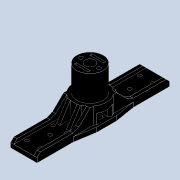
# Autodesk Inventor part: Axis 4 Male Bearing Connector Bracket
Saved by Autodesk Inventor 2022 (Build 260153000, 153)
## iProperties
Created: 2021-12-24
Part Number: Axis 4 Male Bearing Connector Bracket
Material: Generic
Document SubType Name: Modeling
Designer: Coy
Density: 1 g/cm^3
Appearance: Anodized - Black
Author: Coy
Autodesk Inventor part; units mm, degrees
ref_plane "YZ Plane" through (0, 0, 0) normal (1, 0, 0) x (0, 1, 0)
ref_plane "XZ Plane" through (0, 0, 0) normal (0, 1, 0) x (-1, 0, 0)
sketch "Sketch1" plane through (0, 0, 0) normal (0, 1, 0) x (-1, 0, 0)
  line L0 (0, 0) -> (40, 0)
  line L1 (40, 0) -> (40, 200)
  line L2 (40, 200) -> (0, 200)
  line L3 (0, 200) -> (0, 0)
  dimension "d0" = 200
  dimension "d1" = 40
  constraints: 8 end point, 2 parallel, 1 horizontal, 1 perpendicular
  measures "d0" distance of L0.end L1.end
  measures "d1" distance of L0.start L0.end
extrude "Extrusion1" add sketch "Sketch1" along normal blind 7
sketch "Sketch2" plane through (0, 0, 0) normal (0, -1, 0) x (1, 0, 0)
  line L0 (0, 200) -> (0, 0) construction
  line L1 (0, 100) -> (-40, 100) construction
  line L2 (-40, 0) -> (-40, 200) construction
  circle A0 centre (-20, 100) radius 20 construction
  line L3 (-40, 200) -> (0, 200) construction
  line L4 (-20, 200) -> (-20, 0) construction
  line L5 (0, 0) -> (-40, 0) construction
  line L6 (-9.65, 200) -> (-9.65, 0)
  line L7 (-30.35, 200) -> (-30.35, 0)
  line L8 (-9.65, 90) -> (-30.35, 90)
  line L9 (-30.35, 90) -> (-30.35, 23) construction
  line L10 (-30.35, 23) -> (-9.65, 23)
  line L11 (-9.65, 23) -> (-9.65, 90) construction
  line L12 (-9.65, 110) -> (-30.35, 110)
  line L13 (-30.35, 110) -> (-30.35, 177) construction
  line L14 (-30.35, 177) -> (-9.65, 177)
  line L15 (-9.65, 177) -> (-9.65, 110) construction
  line L16 (-9.65, 113.2) -> (-30.35, 113.2) construction
  line L17 (-9.65, 86.8) -> (-30.35, 86.8) construction
  point P0 (-9.65, 177)
  dimension "d19" = 1.25
  dimension "d4" = 40
  dimension "d5" = 10.35
  dimension "d6" = 10.35
  dimension "d7" = 67
  dimension "d8" = 67
  dimension "d9" = 3.2
  dimension "d10" = 3.2
  dimension "d11" = 20
  dimension "d12" = 10
  constraints: 28 end point, 8 point on line, 6 parallel, 5 midpoint, 4 perpendicular, 2 horizontal, 1 centre point
  measures "d4" diameter of A0
  measures "d5" distance between parallel lines of L4 L6
  measures "d6" distance between parallel lines of L4 L7
  measures "d7" distance of L9.end L8.end
  measures "d8" distance between parallel lines of L14 L12
  measures "d9" distance between parallel lines of L12 L16
  measures "d10" distance between parallel lines of L8 L17
  measures "d11" distance between parallel lines of L8 L12
  measures "d12" distance from line of A0.centre L12
extrude "Extrusion2" cut sketch "Sketch2" against normal blind 3.2 contours L6 L12 L7 L14 | L6 L10 L7 L8
sketch "Sketch3" plane through (0, 3.2, 0) normal (0, -1, 0) x (1, 0, 0)
  line L0 (-9.65, 177) -> (-9.65, 110) projected
  line L1 (-30.35, 110) -> (-30.35, 177) projected
  line L2 (-9.65, 110) -> (-30.35, 110)
  line L3 (-30.35, 110) -> (-30.35, 113.3)
  line L4 (-30.35, 113.3) -> (-9.65, 113.3)
  line L5 (-9.65, 113.3) -> (-9.65, 110)
  line L6 (-30.35, 90) -> (-9.65, 90) projected
  line L7 (-30.35, 23) -> (-30.35, 90) projected
  line L8 (-9.65, 90) -> (-30.35, 90)
  line L9 (-30.35, 90) -> (-30.35, 86.7)
  line L10 (-30.35, 86.7) -> (-9.65, 86.7)
  line L11 (-9.65, 86.7) -> (-9.65, 90)
  line L12 (-30.35, 177) -> (-9.65, 177) construction
  line L13 (-20, 177) -> (-20, 110) construction
  line L14 (-20, 90) -> (-20, 23) construction
  line L15 (-9.65, 23) -> (-30.35, 23) construction
  circle A0 centre (-20, 160) radius 2.65
  circle A1 centre (-20, 131) radius 2.65
  circle A2 centre (-20, 69) radius 2.65
  circle A3 centre (-20, 40) radius 2.65
  point P0 (0, 0)
  dimension "d15" = 3.3
  dimension "d16" = 3.3
  dimension "d20" = 5.3
  dimension "d21" = 5.3
  dimension "d22" = 5.3
  dimension "d23" = 5.3
  dimension "d24" = 29
  dimension "d25" = 29
  dimension "d26" = 21
  dimension "d27" = 21
  constraints: 20 end point, 6 point on line, 4 centre point, 4 midpoint, 4 parallel, 2 horizontal, 2 perpendicular
  measures "d15" distance of L2.end L3.end
  measures "d16" distance of L9.end L8.end
  measures "d20" diameter of A0
  measures "d21" diameter of A1
  measures "d22" diameter of A2
  measures "d23" diameter of A3
  measures "d24" distance of A1.centre A0.centre
  measures "d25" distance of A3.centre A2.centre
  measures "d26" distance from line of L2 A1.centre
  measures "d27" distance from line of L6 A2.centre
extrude "Extrusion3" cut sketch "Sketch3" against normal up to next
fillet "Fillet1" radius 1.25 2 edges at (-20, 3.2, 113.3) (-20, 3.2, 86.7)
sketch "Sketch4" plane through (0, 7, 0) normal (0, 1, 0) x (1, 0, 0)
  line L0 (-40, -200) -> (0, -200) construction
  line L1 (-30, -200) -> (-30, 0) construction
  line L2 (-40, 0) -> (-40, -200) construction
  circle A0 centre (-30, -185) radius 2.65
  circle A1 centre (-30, -145.5) radius 2.65
  circle A2 centre (-30, -54.5) radius 2.65
  circle A3 centre (-30, -15) radius 2.65
  line L3 (0, 0) -> (-40, 0) projected
  circle A4 centre (-20, -131) radius 2.65 projected
  circle A5 centre (-20, -69) radius 2.65 projected
  line L4 (-20, -200) -> (-20, 0) construction
  line L5 (0, 0) -> (-40, 0) construction
  line L6 (-10, -200) -> (-10, 0) construction
  line L7 (0, 0) -> (0, -200) construction
  circle A6 centre (-10, -185) radius 2.65
  circle A7 centre (-10, -145.5) radius 2.65
  circle A8 centre (-10, -54.5) radius 2.65
  circle A9 centre (-10, -15) radius 2.65
  dimension "d28" = 10
  dimension "d29" = 5.3
  dimension "d30" = 5.3
  dimension "d31" = 5.3
  dimension "d32" = 5.3
  dimension "d33" = 15
  dimension "d34" = 15
  dimension "d35" = 14.5
  dimension "d36" = 14.5
  constraints: 9 point on line, 8 centre point, 8 end point, 6 symmetric about line, 2 midpoint, 1 vertical, 4 other
  measures "d28" distance between parallel lines of L2 L1
  measures "d29" diameter of A0
  measures "d30" diameter of A1
  measures "d31" diameter of A2
  measures "d32" diameter of A3
  measures "d33" distance from line of L0 A0.centre
  measures "d34" distance from line of L3 A3.centre
  measures "d35" vertical distance of A4.centre A1.centre
  measures "d36" vertical distance of A5.centre A2.centre
extrude "Extrusion4" cut sketch "Sketch4" against normal up to next contours A0 | A1 | A2 | A3 | A6 | A7 | A8 | A9
sketch "Sketch5" plane through (0, 7, 0) normal (0, 1, 0) x (1, 0, 0)
  circle A0 centre (-30, -145.5) radius 2.65 projected
  circle A1 centre (-30, -15) radius 2.65 projected
  circle A2 centre (-10, -54.5) radius 2.65 projected
  circle A3 centre (-10, -185) radius 2.65 projected
  circle A4 centre (-10, -145.5) radius 2.65 projected
  circle A5 centre (-10, -15) radius 2.65 projected
  circle A6 centre (-30, -54.5) radius 2.65 projected
  circle A7 centre (-30, -185) radius 2.65 projected
  circle A8 centre (-20, -69) radius 2.65 projected
  line L0 (-30.35, -90) -> (-30.35, -86.7) projected
  line L1 (-30.35, -86.7) -> (-9.65, -86.7) projected
  line L2 (-9.65, -86.7) -> (-9.65, -90) projected
  line L3 (-9.65, -90) -> (-30.35, -90) projected
  circle A9 centre (-20, -131) radius 2.65 projected
  circle A10 centre (-20, -40) radius 2.65 projected
  line L4 (-9.65, -113.3) -> (-30.35, -113.3) projected
  line L5 (-30.35, -113.3) -> (-30.35, -110) projected
  line L6 (-30.35, -110) -> (-9.65, -110) projected
  line L7 (-9.65, -110) -> (-9.65, -113.3) projected
  circle A11 centre (-20, -160) radius 2.65 projected
  line L8 (-40, 0) -> (-40, -200) projected
  line L9 (-40, -200) -> (0, -200) projected
  line L10 (0, -200) -> (0, 0) projected
  line L11 (0, 0) -> (-40, 0) projected
  line L12 (-40, -200) -> (0, -200) construction
  line L13 (-20, -200) -> (-20, 0) construction
  line L14 (0, 0) -> (-40, 0) construction
  circle A12 centre (-20, -100) radius 20
  line L15 (-40, 0) -> (-40, -200) projected
  circle A13 centre (-20, -100) radius 7.5
  dimension "d39" = 15
  constraints: 3 midpoint, 2 centre point, 2 end point, 1 coincident, 1 tangent
  measures "d39" diameter of A13
extrude "Extrusion5" add sketch "Sketch5" along normal blind 64 contours A12
sketch "Sketch6" plane through (0, 7, 0) normal (0, 1, 0) x (1, 0, 0)
  circle A0 centre (-20, -69) radius 2.65 construction
  circle A1 centre (-20, -69) radius 5 construction
  circle A2 centre (-20, -100) radius 20 projected
  circle A3 centre (-20, -100) radius 25
  point P0 (0, 0)
  dimension "d42" = 10
  dimension "d43" = 50
  constraints: 2 centre point, 2 coincident
  measures "d42" diameter of A1
  measures "d43" diameter of A3
extrude "Extrusion6" add sketch "Sketch6" along normal blind 25
sketch "Sketch7" plane through (-20, 71, 100) normal (0, 1, 0) x (1, 0, 0)
  line L0 (-20, 15) -> (-20, -15) construction
  line L1 (-20, 0) -> (20, 0) construction
  circle A0 centre (0, 0) radius 20 construction
  circle A1 centre (-13.75, 0) radius 2.75
  circle A2 centre (13.75, 0) radius 2.75
  circle A3 centre (-13.75, 0) radius 5 construction
  circle A4 centre (13.75, 0) radius 5 construction
  point P0 (20, 100)
  dimension "d46" = 5.5
  dimension "d47" = 5.5
  dimension "d48" = 6.25
  dimension "d49" = 10
  dimension "d50" = 10
  dimension "d51" = 6.25
  constraints: 4 centre point, 2 coincident, 2 end point, 2 point on line, 1 horizontal, 1 midpoint, 1 point on circle
  measures "d46" diameter of A1
  measures "d47" diameter of A2
  measures "d48" distance of L1.start A1.centre
  measures "d49" diameter of A3
  measures "d50" diameter of A4
  measures "d51" distance of L1.end A2.centre
extrude "Extrusion7" cut sketch "Sketch7" against normal up to next
sketch "Sketch8" plane through (0, 0, 0) normal (0, -1, 0) x (1, 0, 0)
  circle A0 centre (-6.25, 100) radius 2.75 projected
  circle A1 centre (-33.75, 100) radius 2.75 projected
  line L0 (-2.25, 97.6906) -> (-6.25, 95.3812)
  line L1 (-6.25, 95.3812) -> (-10.25, 97.6906)
  line L2 (-10.25, 97.6906) -> (-10.25, 102.3094)
  line L3 (-10.25, 102.3094) -> (-6.25, 104.6188)
  line L4 (-6.25, 104.6188) -> (-2.25, 102.3094)
  line L5 (-2.25, 102.3094) -> (-2.25, 97.6906)
  line L6 (-29.75, 97.6906) -> (-33.75, 95.3812)
  line L7 (-33.75, 95.3812) -> (-37.75, 97.6906)
  line L8 (-37.75, 97.6906) -> (-37.75, 102.3094)
  line L9 (-37.75, 102.3094) -> (-33.75, 104.6188)
  line L10 (-33.75, 104.6188) -> (-29.75, 102.3094)
  line L11 (-29.75, 102.3094) -> (-29.75, 97.6906)
  point P0 (0, 0)
  dimension "d54" = 8
  dimension "d55" = 8
  constraints: 24 end point, 2 coincident, 26 other
  measures "d54" distance between parallel lines of L2 L5
  measures "d55" distance between parallel lines of L8 L11
extrude "Extrusion8" cut sketch "Sketch8" against normal blind 51
sketch "Sketch9" plane through (0, 0, 0) normal (0, -1, 0) x (1, 0, 0)
  line L0 (-37.75, 102.3094) -> (-33.75, 104.6188) projected
  line L1 (-33.75, 104.6188) -> (-29.75, 102.3094) projected
  line L2 (-29.75, 102.3094) -> (-29.75, 97.6906) projected
  line L3 (-29.75, 97.6906) -> (-33.75, 95.3812) projected
  line L4 (-33.75, 95.3812) -> (-37.75, 97.6906) projected
  line L5 (-37.75, 97.6906) -> (-37.75, 102.3094) projected
  line L6 (-10.25, 102.3094) -> (-6.25, 104.6188) projected
  line L7 (-6.25, 104.6188) -> (-2.25, 102.3094) projected
  line L8 (-2.25, 102.3094) -> (-2.25, 97.6906) projected
  line L9 (-2.25, 97.6906) -> (-6.25, 95.3812) projected
  line L10 (-6.25, 95.3812) -> (-10.25, 97.6906) projected
  line L11 (-10.25, 97.6906) -> (-10.25, 102.3094) projected
  line L12 (-40, 0) -> (-40, 200) projected
  line L13 (0, 0) -> (-40, 0) projected
  line L14 (0, 200) -> (0, 0) projected
  line L15 (-40, 200) -> (0, 200) projected
  arc A0 (-9.65, 51.8732) -> (-9.65, 57.1268) centre (-10, 54.5) ccw projected
  line L16 (-9.65, 51.8732) -> (-9.65, 23) projected
  line L17 (-9.65, 23) -> (-30.35, 23) projected
  line L18 (-30.35, 23) -> (-30.35, 51.8732) projected
  arc A1 (-30.35, 57.1268) -> (-30.35, 51.8732) centre (-30, 54.5) ccw projected
  line L19 (-30.35, 57.1268) -> (-30.35, 90) projected
  line L20 (-30.35, 90) -> (-9.65, 90) projected
  line L21 (-9.65, 90) -> (-9.65, 57.1268) projected
  circle A2 centre (-30, 185) radius 2.65 projected
  circle A3 centre (-10, 15) radius 2.65 projected
  circle A4 centre (-10, 185) radius 2.65 projected
  circle A5 centre (-30, 15) radius 2.65 projected
  arc A6 (-30.35, 148.1268) -> (-30.35, 142.8732) centre (-30, 145.5) ccw projected
  line L22 (-30.35, 148.1268) -> (-30.35, 177) projected
  line L23 (-30.35, 177) -> (-9.65, 177) projected
  line L24 (-9.65, 177) -> (-9.65, 148.1268) projected
  arc A7 (-9.65, 142.8732) -> (-9.65, 148.1268) centre (-10, 145.5) ccw projected
  line L25 (-9.65, 142.8732) -> (-9.65, 110) projected
  line L26 (-9.65, 110) -> (-30.35, 110) projected
  line L27 (-30.35, 110) -> (-30.35, 142.8732) projected
  line L28 (0, 115) -> (0, 85) projected
  arc A8 (0, 85) -> (0, 115) centre (-20, 100) ccw projected
  line L29 (-40, 85) -> (-40, 115) projected
  arc A9 (-40, 115) -> (-40, 85) centre (-20, 100) ccw projected
  line L30 (5, 115) -> (-45, 115)
  line L31 (-45, 115) -> (-45, 85)
  line L32 (-45, 85) -> (5, 85)
  line L33 (5, 85) -> (5, 115)
  line L34 (5, 115) -> (0, 145.5)
  line L35 (0, 200) -> (0, 0) projected
  line L36 (-45, 115) -> (-40, 145.5)
  line L37 (-40, 0) -> (-40, 200) projected
  line L38 (-45, 85) -> (-40, 54.5)
  line L39 (5, 85) -> (0, 54.5)
  constraints: 16 end point, 4 parallel, 4 point on line, 1 horizontal, 1 perpendicular
extrude "Extrusion9" add sketch "Sketch9" against normal up to surface (7 mm away) contours L38 L32 L12 | A9 L12 | L32 L31 A9 | L14 L32 L39 | L30 L36 L12 | A9 L31 L30 | L14 A8 | A8 L33 L32 | L30 L33 A8 | L14 L34 L30
sketch "Sketch10" plane through (0, 7, 0) normal (0, 1, 0) x (1, 0, 0)
  arc A0 (-45, -100) -> (5, -100) centre (-20, -100) ccw projected
  line L0 (-45, -115) -> (-45, -100) projected
  line L1 (-40, -145.5) -> (-45, -115) projected
  line L2 (-40, -145.5) -> (-40, -200) projected
  line L3 (-40, -200) -> (0, -200) projected
  line L4 (0, -200) -> (0, -145.5) projected
  line L5 (5, -115) -> (0, -145.5) projected
  line L6 (5, -100) -> (5, -115) projected
  circle A1 centre (-20, -160) radius 2.65 projected
  circle A2 centre (-20, -131) radius 2.65 projected
  circle A3 centre (-30, -185) radius 2.65 projected
  circle A4 centre (-10, -145.5) radius 2.65 projected
  circle A5 centre (-10, -185) radius 2.65 projected
  circle A6 centre (-30, -145.5) radius 2.65 projected
  circle A7 centre (-20, -40) radius 2.65 projected
  circle A8 centre (-20, -69) radius 2.65 projected
  circle A9 centre (-30, -54.5) radius 2.65 projected
  circle A10 centre (-10, -15) radius 2.65 projected
  circle A11 centre (-10, -54.5) radius 2.65 projected
  circle A12 centre (-30, -15) radius 2.65 projected
  arc A13 (5, -100) -> (-45, -100) centre (-20, -100) ccw projected
  line L7 (5, -85) -> (5, -100) projected
  line L8 (0, -54.5) -> (5, -85) projected
  line L9 (0, -54.5) -> (0, 0) projected
  line L10 (0, 0) -> (-40, 0) projected
  line L11 (-40, 0) -> (-40, -54.5) projected
  line L12 (-45, -85) -> (-40, -54.5) projected
  line L13 (-45, -100) -> (-45, -85) projected
  line L14 (-65.195, -100) -> (40.5448, -100) construction
  circle A14 centre (-10, -145.5) radius 5 construction
  line L15 (5, -115) -> (0, -145.5) projected
  line L16 (0, -145.5) -> (-5, -145.5)
  line L17 (-5, -145.5) -> (-5, -120)
  arc A15 (-45, -100) -> (5, -100) centre (-20, -100) ccw projected
  line L18 (0, -200) -> (0, -145.5) projected
  line L19 (0, -145.5) -> (0, -115)
  line L20 (-40, -200) -> (0, -200) construction
  line L21 (-20, -200) -> (-20, 0) construction
  line L22 (0, 0) -> (-40, 0) construction
  circle A16 centre (-20, -131) radius 2.65 construction
  circle A17 centre (-20, -131) radius 5 construction
  line L23 (-15, -124.4949) -> (-15, -140.5)
  line L24 (-15, -140.5) -> (-10, -140.5)
  line L25 (-10, -140.5) -> (-10, -122.9129)
  line L26 (-40, -145.5) -> (-35, -145.5)
  line L27 (-35, -145.5) -> (-35, -120)
  line L28 (-40, -145.5) -> (-40, -115)
  line L29 (-25, -124.4949) -> (-25, -140.5)
  line L30 (-25, -140.5) -> (-30, -140.5)
  line L31 (-30, -140.5) -> (-30, -122.9129)
  line L32 (0, -54.5) -> (-5, -54.5)
  line L33 (-5, -54.5) -> (-5, -80)
  line L34 (0, -54.5) -> (0, -85)
  line L35 (-15, -75.5051) -> (-15, -59.5)
  line L36 (-15, -59.5) -> (-10, -59.5)
  line L37 (-10, -59.5) -> (-10, -77.0871)
  line L38 (-25, -75.5051) -> (-25, -59.5)
  line L39 (-25, -59.5) -> (-30, -59.5)
  line L40 (-30, -59.5) -> (-30, -77.0871)
  line L41 (-35, -54.5) -> (-35, -80)
  line L42 (-40, -54.5) -> (-35, -54.5)
  line L43 (-40, -54.5) -> (-40, -85)
  dimension "d60" = 10
  dimension "d61" = 5
  dimension "d62" = 10
  dimension "d63" = 5
  constraints: 52 end point, 21 symmetric about line, 6 point on circle, 2 centre point, 2 coincident, 2 midpoint, 2 perpendicular, 1 collinear, 1 vertical
  measures "d60" diameter of A14
  measures "d61" distance of L4.end L16.end
  measures "d62" diameter of A17
  measures "d63" distance of L23.end L24.end
extrude "Extrusion10" add sketch "Sketch10" along normal blind 25 contours A0 L27 L26 L28 | L43 L42 L41 A13 | A0 L29 L30 L31 | L40 L39 L38 A13 | A0 L25 L24 L23 | L16 L17 A0 L19 | L35 L36 L37 A13 | L34 A13 L33 L32
chamfer "Chamfer1" distance 25.5 distance2 25 1 edges at (-2.5, 32, 145.5) measured on face at (-38.3333, 32, 126.8333)
chamfer "Chamfer2" distance 25.5 distance2 25 1 edges at (-37.5, 32, 145.5) measured on face at (-38.3333, 32, 126.8333)
chamfer "Chamfer3" distance 25.5 distance2 25 1 edges at (-2.5, 32, 54.5) measured on face at (-1.6667, 32, 73.1667)
chamfer "Chamfer4" distance 25.5 distance2 25 1 edges at (-37.5, 32, 54.5) measured on face at (-38.3333, 32, 73.1667)
chamfer "Chamfer5" distance 16 distance2 25 1 edges at (-12.5, 32, 140.5) measured on face at (-28.3333, 32, 70.6974)
chamfer "Chamfer6" distance 16 distance2 25 1 edges at (-27.5, 32, 140.5) measured on face at (-28.3333, 32, 70.6974)
chamfer "Chamfer7" distance 16 distance2 25 1 edges at (-12.5, 32, 59.5) measured on face at (-28.3333, 32, 70.6974)
chamfer "Chamfer8" distance 16 distance2 25 1 edges at (-27.5, 32, 59.5) measured on face at (-28.3333, 32, 70.6974)
ref_plane "Work Plane1" through (0, 12, 0) normal (0, 1, 0) x (1, 0, 0)
sketch "Sketch11" plane through (0, 12, 0) normal (0, 1, 0) x (1, 0, 0)
  circle A0 centre (-30, -185) radius 2.65 construction
  circle A1 centre (-30, -185) radius 5 construction
  line L0 (-40, -145.5) -> (-40, -200) projected
  line L1 (-35, -120) -> (-35, -145.5) projected
  line L2 (-40, -200) -> (-35, -200)
  line L3 (-35, -200) -> (-35, -140)
  line L4 (-35, -140) -> (-40, -140)
  line L5 (-40, -140) -> (-40, -200)
  line L6 (-40, -200) -> (0, -200) construction
  circle A2 centre (-20, -100) radius 7.5 construction
  line L7 (-20, -200) -> (-20, -100) construction
  line L8 (-20, -100) -> (-45, -100) construction
  arc A3 (-40, -85) -> (-40, -115) centre (-20, -100) ccw construction
  line L9 (0, -145.5) -> (0, -200)
  line L10 (0, -200) -> (-5, -200)
  line L11 (-5, -200) -> (-5, -140)
  line L12 (-5, -140) -> (0, -140)
  line L13 (0, -140) -> (0, -200)
  circle A4 centre (-30, -15) radius 2.65 construction
  circle A5 centre (-30, -15) radius 5 construction
  line L14 (-40, -54.5) -> (-40, 0)
  line L15 (-40, 0) -> (-35, 0)
  line L16 (-35, 0) -> (-35, -60)
  line L17 (-35, -60) -> (-40, -60)
  line L18 (-40, -60) -> (-40, 0)
  line L19 (-40, 0) -> (0, 0) construction
  line L20 (0, -54.5) -> (0, 0)
  line L21 (0, 0) -> (-5, 0)
  line L22 (-5, 0) -> (-5, -60)
  line L23 (-5, -60) -> (0, -60)
  line L24 (0, -60) -> (0, 0)
  point P0 (0, 0)
  point P1 (-5, -145.5)
  point P2 (-35, -54.5)
  point P3 (-20, 0)
  point P4 (-5, -54.5)
  dimension "d91" = 10
  dimension "d92" = 60
  constraints: 44 end point, 20 symmetric about line, 3 centre point, 2 coincident, 2 parallel, 2 perpendicular, 1 horizontal, 1 midpoint, 1 point on circle, 1 point on line, 1 vertical, 2 other
  measures "d91" diameter of A1
  measures "d92" distance of L3.end L2.end
extrude "Extrusion11" add sketch "Sketch11" against normal up to next
chamfer "Chamfer9" distance 5 angle 45 8 edges at (-37.5, 12, 200) (-2.5, 12, 200) (-37.5, 12, 0) (-2.5, 12, 0) (-2.5, 12, 140.4005) (-37.5, 12, 140.4005) (-37.5, 12, 59.5995) (-2.5, 12, 59.5995)
sketch "Sketch12" plane through (5, 0, 115) normal (1, 0, 0) x (0, 0, -1)
  line L0 (7.5, 71) -> (22.5, 71) projected
  line L1 (22.5, 7) -> (7.5, 7) projected
  line L2 (22.5, 7) -> (7.5, 7) projected
  line L3 (7.5, 71) -> (7.5, 7) projected
  line L4 (22.5, 7) -> (7.5, 7)
  line L5 (7.5, 7) -> (7.5, 22)
  line L6 (7.5, 22) -> (22.5, 22)
  line L7 (22.5, 22) -> (22.5, 7)
  point P0 (115, 0)
  dimension "d98" = 15
  constraints: 8 end point, 2 parallel, 1 horizontal, 1 perpendicular, 1 point on line
  measures "d98" distance of L4.end L5.end
extrude "Extrusion12" cut sketch "Sketch12" against normal through all
fillet "Fillet2" radius 3 4 edges at (-43.8485, 14.5, 107.5) (3.8485, 14.5, 107.5) (-43.8485, 14.5, 92.5) (3.8485, 14.5, 92.5)
equation "\"d6\" = d5"
equation "\"d8\" = d7"
equation "\"d10\" = d9"
equation "\"d12\" = 0.5 * d11"
equation "\"d21\" = d20"
equation "\"d22\" = d20"
equation "\"d23\" = d20"
equation "\"d25\" = d24"
equation "\"d27\" = d26"
equation "\"d30\" = d29"
equation "\"d31\" = d29"
equation "\"d32\" = d29"
equation "\"d36\" = d35"
equation "\"d37\" = d31"
equation "\"d50\" = d49"
equation "\"d51\" = d48"
equation "\"d55\" = d54"
body "Solid1"
